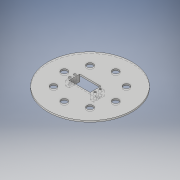
# Autodesk Inventor part: bottom_platform
Saved by Autodesk Inventor 2018 (Build 220112000, 112)
## iProperties
Created: 2018-04-16
Part Number: bottom_platform
Material: Generic
Document SubType Name: Modeling
Designer: scwu
Density: 1 g/cm^3
Appearance: Default
Author: scwu
Autodesk Inventor part; units mm, degrees
ref_plane "YZ Plane" through (0, 0, 0) normal (1, 0, 0) x (0, 1, 0)
ref_plane "XZ Plane" through (0, 0, 0) normal (0, 1, 0) x (-1, 0, 0)
ref_plane "XY Plane" through (0, 0, 0) normal (0, 0, 1) x (1, 0, 0)
sketch "Sketch9" plane through (0, 0, 0) normal (0, 1, 0) x (-1, 0, 0)
  circle A0 centre (0, 0) radius 81.6944
  dimension "d64" = 163.3888
  constraints: 1 centre point, 1 coincident
  measures "d64" diameter of A0
extrude "Extrusion4" add sketch "Sketch9" along normal blind 3
derived "feedback_servo.ipt"
sketch "Sketch6" plane through (-20, 0, 10) normal (0, -1, 0) x (1, 0, 0)
  line L0 (0, 0) -> (0, -20) construction
  line L1 (0, -10) -> (40, -10) construction
  line L2 (40, -20) -> (40, 0) construction
  line L3 (40, 0) -> (0, 0) construction
  line L4 (20, 0) -> (20, -20) construction
  line L5 (0, -20) -> (40, -20) construction
  line L6 (40, 0) -> (0, 0) construction
  line L7 (0, 0) -> (0, -20) construction
  line L8 (0, -20) -> (40, -20) construction
  line L9 (40, -20) -> (40, 0) construction
  circle A0 centre (29.7, -10) radius 2.8
  circle A1 centre (-4.75, -5) radius 2
  circle A2 centre (-4.75, -15) radius 2
  circle A3 centre (44.75, -15) radius 2
  circle A4 centre (44.75, -5) radius 2
  line L10 (-7.4, -10.75) -> (0, -10.75)
  line L11 (0, -9.25) -> (-7.4, -9.25)
  line L12 (40, -10.75) -> (47.4, -10.75)
  line L13 (47.4, -9.25) -> (40, -9.25)
  line L14 (40, -20) -> (40, 0)
  line L15 (47.4, -20) -> (47.4, 0)
  line L16 (40, 0) -> (47.4, 0)
  circle A5 centre (44.75, -15) radius 2
  circle A6 centre (44.75, -5) radius 2
  line L17 (47.4, -20) -> (47.4, 0)
  line L18 (40, 0) -> (47.4, 0)
  line L19 (40, -20) -> (40, 0)
  line L20 (47.4, -20) -> (40, -20)
  circle A7 centre (-4.75, -15) radius 2
  circle A8 centre (-4.75, -5) radius 2
  line L21 (0, -20) -> (0, 0)
  line L22 (-7.4, 0) -> (0, 0)
  line L23 (-7.4, -20) -> (-7.4, 0)
  line L24 (0, -20) -> (-7.4, -20)
  point P0 (20, -10)
sketch "Sketch18" plane through (0, 0, 0) normal (0, -1, 0) x (1, 0, 0)
  line L0 (-29.7, 10) -> (-29.7, -10) construction
  line L1 (-29.7, 0) -> (10.3, 0) construction
  line L2 (10.3, -10) -> (10.3, 10) construction
  line L3 (10.3, 10) -> (-29.7, 10) construction
  line L4 (-9.7, 10) -> (-9.7, -10) construction
  line L5 (-29.7, -10) -> (10.3, -10) construction
  line L6 (10.3, 10) -> (-29.7, 10) construction
  line L7 (-29.7, 10) -> (-29.7, -10) construction
  line L8 (-29.7, -10) -> (10.3, -10) construction
  line L9 (10.3, -10) -> (10.3, 10) construction
  circle A0 centre (0, 0) radius 2.8
  circle A1 centre (-34.45, 5) radius 2
  circle A2 centre (-34.45, -5) radius 2
  circle A3 centre (15.05, -5) radius 2
  circle A4 centre (15.05, 5) radius 2
  line L10 (-37.1, -0.75) -> (-29.7, -0.75)
  line L11 (-29.7, 0.75) -> (-37.1, 0.75)
  line L12 (10.3, -0.75) -> (17.7, -0.75)
  line L13 (17.7, 0.75) -> (10.3, 0.75)
  line L14 (10.3, -10) -> (10.3, 10)
  line L15 (17.7, -10) -> (17.7, 10)
  line L16 (10.3, 10) -> (17.7, 10)
  circle A5 centre (15.05, -5) radius 2
  circle A6 centre (15.05, 5) radius 2
  line L17 (17.7, -10) -> (17.7, 10)
  line L18 (10.3, 10) -> (17.7, 10)
  line L19 (10.3, -10) -> (10.3, 10)
  line L20 (17.7, -10) -> (10.3, -10)
  circle A7 centre (-34.45, -5) radius 2
  circle A8 centre (-34.45, 5) radius 2
  line L21 (-29.7, -10) -> (-29.7, 10)
  line L22 (-37.1, 10) -> (-29.7, 10)
  line L23 (-37.1, -10) -> (-37.1, 10)
  line L24 (-29.7, -10) -> (-37.1, -10)
  point P0 (0, 0)
  point P1 (-9.7, 0)
  constraints: 50 end point, 9 centre point
sketch "Sketch19" plane through (0, 0, 0) normal (0, -1, 0) x (1, 0, 0)
  line L0 (10.8, 10.5) -> (-30.2, 10.5)
  line L1 (-30.2, 10.5) -> (-30.2, -10.5)
  line L2 (-30.2, -10.5) -> (10.8, -10.5)
  line L3 (10.8, -10.5) -> (10.8, 10.5)
  line L4 (10.8, 10.5) -> (-30.2, -10.5) construction
  line L5 (-30.2, 10.5) -> (10.8, -10.5) construction
  line L6 (-30.2, 10.5) -> (-37.2, 10.5)
  line L7 (-37.2, 10.5) -> (-37.2, -10.5)
  line L8 (-37.2, -10.5) -> (-30.2, -10.5)
  line L9 (-30.2, -10.5) -> (-30.2, 10.5)
  line L10 (10.8, 10.5) -> (17.8, 10.5)
  line L11 (17.8, 10.5) -> (17.8, -10.5)
  line L12 (17.8, -10.5) -> (10.8, -10.5)
  line L13 (10.8, -10.5) -> (10.8, 10.5)
  line L14 (-30.2, 0.75) -> (-37.2, 0.75)
  line L15 (-37.2, 0.75) -> (-37.2, -0.75)
  line L16 (-37.2, -0.75) -> (-30.2, -0.75)
  line L17 (-30.2, -0.75) -> (-30.2, 0.75)
  line L18 (10.8, 0.75) -> (17.8, 0.75)
  line L19 (17.8, 0.75) -> (17.8, -0.75)
  line L20 (17.8, -0.75) -> (10.8, -0.75)
  line L21 (10.8, -0.75) -> (10.8, 0.75)
  point P0 (0, 0)
  point P1 (-9.7, 0)
  point P2 (-29.7, -0.75)
  point P3 (-29.7, 0.75)
  point P4 (10.3, -0.75)
  point P5 (10.3, 0.75)
  dimension "d94" = 41
  dimension "d95" = 21
  dimension "d98" = 7
  dimension "d99" = 7
  constraints: 44 end point, 10 parallel, 7 point on line, 5 horizontal, 5 perpendicular, 2 midpoint
  measures "d94" distance of L2.end L1.end
  measures "d95" distance of L1.end L0.end
  measures "d98" distance of L8.end L7.end
  measures "d99" distance of L11.end L12.end
extrude "Extrusion10" cut sketch "Sketch19" against normal up to next contours L3 L2 L1 L0
extrude "Extrusion11" add sketch "Sketch19" along normal blind 10 contours L10 L11 L18 L3 | L1 L14 L7 L6 | L20 L11 L12 L3 | L1 L8 L7 L16
extrude "Extrusion12" cut sketch "Sketch18" along normal through all both and the other way through all contours A1 | A2 | A3 | A4
extrude "Extrusion13" add sketch "Sketch19" along normal blind 8 contours L18 L11 L20 L3 | L1 L16 L7 L14
sketch "Sketch20" plane through (0, 3, 0) normal (0, 1, 0) x (1, 0, 0)
  circle A0 centre (50, 0) radius 6
  circle A1 centre (35.3553, 35.3553) radius 6
  circle A2 centre (0, 50) radius 6
  circle A3 centre (-35.3553, 35.3553) radius 6
  circle A4 centre (-50, 0) radius 6
  circle A5 centre (-35.3553, -35.3553) radius 6
  circle A6 centre (0, -50) radius 6
  circle A7 centre (35.3553, -35.3553) radius 6
  point P0 (0, 0)
  dimension "d106" = 12
  dimension "d109" = 360
  constraints: 8 centre point, 17 other
  measures "d106" diameter of A0
extrude "Extrusion14" cut sketch "Sketch20" against normal up to next
body "Solid1"
